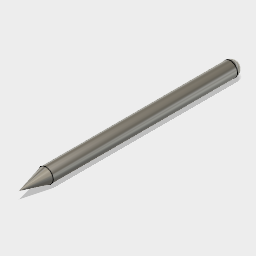
222 (Autodesk Fusion 360 design; units mm, degrees)
Autodesk Fusion 360 part; units mm, degrees
cylinder "圆柱体基本要素1" add diameter 8 height 100 placed x (1, 0, 0) y (0, 1, 0) z (0, 0, 1) at (0, 20, 0) makes body 1
sphere "球体基本要素1" add diameter 8 placed x (1, 0, 0) y (0, 1, 0) z (0, 0, 1) at (30, 20, 0) separate body makes body 2
move_body "对齐1" bodies 2 to x (1, 0, 0) y (0, 1, 0) z (0, 0, 1) at (-26, 0, 0)
move_face "MoveFace1" to x (1, 0, 0) y (0, 1, 0) z (0, 0, 1) at (-3.3109, 0.0975, -0.4969) 2 faces at (7.7923, 20.9455, -0.8511) (1.6151, 19.2874, 0) on bodies 1 2
move_body "对齐2" bodies 1 to x (1, 0, 0) y (0, 1, 0) z (0, 0, 1) at (4.6891, 0.0975, 0)
move_body "对齐3" bodies 1 to x (1, 0, 0) y (0, 1, 0) z (0, 0, 1) at (-4, 0, 0)
sketch "草图4" plane through (0, 0, 0) normal (0, 1, 0) x (1, 0, 0)
  line L0 (50, 0) -> (46, 0)
  line L1 (46, 0) -> (46, -15)
  line L2 (46, -15) -> (50, 0)
revolve "旋转2" add sketch "草图4" angle 360 about axis through (46, 0, 0) along (0, 0, 1) separate body makes body 3
move_body "对齐4" bodies 3 to x (1, 0, 0) y (0, 1, 0) z (0, 0, 1) at (-45.3109, 20.0975, 100)
combine "合并1" operation add target body 3 tool bodies 1 2
move_body "移动1" bodies 3 to x (1, 0, 0) y (0, 1, 0) z (0, 0, 1) at (0, -21.2028, 4.9781)
